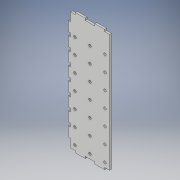
# Autodesk Inventor part: 2 binnen zijplaat
Saved by Autodesk Inventor 2019 (Build 230136000, 136)
## iProperties
Created: 2021-01-09
Part Number: 2 binnen zijplaat
Material: Generic
Document SubType Name: Sheet Metal
Designer: Stefan
Density: 1 g/cm^3
Sheet Metal Rule: Default_mm
Appearance: Default
Author: Stefan
Autodesk Inventor part; units mm, degrees
ref_plane "YZ Plane" through (0, 0, 0) normal (1, 0, 0) x (0, 1, 0)
ref_plane "XZ Plane" through (0, 0, 0) normal (0, 1, 0) x (-1, 0, 0)
ref_plane "XY Plane" through (0, 0, 0) normal (0, 0, 1) x (1, 0, 0)
sketch "Sketch1" plane through (0, 0, 0) normal (0, 0, 1) x (1, 0, 0)
  line L0 (-30, -90.5) -> (30, -90.5)
  line L1 (30, -90.5) -> (30, 90.5)
  line L2 (30, 90.5) -> (-30, 90.5)
  line L3 (-30, 90.5) -> (-30, -90.5)
  line L4 (-30, -90.5) -> (30, 90.5) construction
  line L5 (30, -90.5) -> (-30, 90.5) construction
  circle A0 centre (-23, 60.5) radius 2
  circle A1 centre (-23, 36.5) radius 2
  circle A2 centre (-23, 12.5) radius 2
  circle A3 centre (-23, -11.5) radius 2
  circle A4 centre (-23, -35.5) radius 2
  circle A5 centre (-23, -59.5) radius 2
  circle A6 centre (-23, -83.5) radius 2
  circle A7 centre (0, 60.5) radius 2
  circle A8 centre (0, 36.5) radius 2
  circle A9 centre (0, 12.5) radius 2
  circle A10 centre (0, -11.5) radius 2
  circle A11 centre (0, -35.5) radius 2
  circle A12 centre (0, -59.5) radius 2
  circle A13 centre (0, -83.5) radius 2
  circle A14 centre (23, 60.5) radius 2
  circle A15 centre (23, 36.5) radius 2
  circle A16 centre (23, 12.5) radius 2
  circle A17 centre (23, -11.5) radius 2
  circle A18 centre (23, -35.5) radius 2
  circle A19 centre (23, -59.5) radius 2
  circle A20 centre (23, -83.5) radius 2
  point P0 (0, 0)
  dimension "d0" = 60
  dimension "d1" = 181
  dimension "d2" = 4
  dimension "d3" = 30
  dimension "d6" = 24
  dimension "d9" = 23
  dimension "d12" = 7
  constraints: 21 centre point, 12 end point, 2 horizontal, 2 midpoint, 2 parallel, 1 perpendicular, 1 vertical, 40 other
  measures "d0" distance of L2.end L1.end
  measures "d1" distance of L1.end L0.end
  measures "d2" diameter of A0
  measures "d3" distance from line of A0.centre L2
  measures "d6" distance of A0.centre A1.centre
  measures "d9" distance of A0.centre A7.centre
  measures "d12" distance from line of L3 A0.centre
extrude "Extrusion1" add sketch "Sketch1" along normal blind 3
sketch "Sketch2" plane through (0, 0, 3) normal (0, 0, 1) x (1, 0, 0)
  line L0 (-30, 90.5) -> (-30, -90.5) projected
  line L1 (-30, 77.5) -> (-33, 77.5)
  line L2 (-33, 77.5) -> (-33, 62.5)
  line L3 (-33, 62.5) -> (-30, 62.5)
  line L4 (-30, 62.5) -> (-30, 77.5)
  line L5 (-30, 57.5) -> (-33, 57.5)
  line L6 (-33, 57.5) -> (-33, 42.5)
  line L7 (-33, 42.5) -> (-30, 42.5)
  line L8 (-30, 42.5) -> (-30, 57.5)
  line L9 (-30, 37.5) -> (-33, 37.5)
  line L10 (-33, 37.5) -> (-33, 22.5)
  line L11 (-33, 22.5) -> (-30, 22.5)
  line L12 (-30, 22.5) -> (-30, 37.5)
  line L13 (-30, 17.5) -> (-33, 17.5)
  line L14 (-33, 17.5) -> (-33, 2.5)
  line L15 (-33, 2.5) -> (-30, 2.5)
  line L16 (-30, 2.5) -> (-30, 17.5)
  line L17 (-30, -2.5) -> (-33, -2.5)
  line L18 (-33, -2.5) -> (-33, -17.5)
  line L19 (-33, -17.5) -> (-30, -17.5)
  line L20 (-30, -17.5) -> (-30, -2.5)
  line L21 (-30, -22.5) -> (-33, -22.5)
  line L22 (-33, -22.5) -> (-33, -37.5)
  line L23 (-33, -37.5) -> (-30, -37.5)
  line L24 (-30, -37.5) -> (-30, -22.5)
  line L25 (-30, -42.5) -> (-33, -42.5)
  line L26 (-33, -42.5) -> (-33, -57.5)
  line L27 (-33, -57.5) -> (-30, -57.5)
  line L28 (-30, -57.5) -> (-30, -42.5)
  line L29 (-30, -62.5) -> (-33, -62.5)
  line L30 (-33, -62.5) -> (-33, -77.5)
  line L31 (-33, -77.5) -> (-30, -77.5)
  line L32 (-30, -77.5) -> (-30, -62.5)
  point P0 (0, 0)
  dimension "d15" = 3
  dimension "d16" = 15
  dimension "d17" = 13
  dimension "d20" = 20
  constraints: 64 end point, 2 parallel, 1 horizontal, 1 perpendicular, 1 point on line, 1 vertical, 56 other
  measures "d15" distance of L3.end L2.end
  measures "d16" distance of L2.end L1.end
  measures "d17" distance from line of L0.start L1
  measures "d20" distance of L1.start L5.start
extrude "Extrusion2" add sketch "Sketch2" against normal blind 3
sketch "Sketch3" plane through (0, 0, 3) normal (0, 0, 1) x (1, 0, 0)
  line L0 (30, 90.5) -> (-30, 90.5) projected
  line L1 (-22.5, 90.5) -> (-7.5, 90.5)
  line L2 (-7.5, 90.5) -> (-7.5, 93.5)
  line L3 (-7.5, 93.5) -> (-22.5, 93.5)
  line L4 (-22.5, 93.5) -> (-22.5, 90.5)
  line L5 (-22.5, -93.5) -> (-7.5, -93.5)
  line L6 (-7.5, -93.5) -> (-7.5, -90.5)
  line L7 (-7.5, -90.5) -> (-22.5, -90.5)
  line L8 (-22.5, -90.5) -> (-22.5, -93.5)
  line L9 (7.5, 90.5) -> (22.5, 90.5)
  line L10 (22.5, 90.5) -> (22.5, 93.5)
  line L11 (22.5, 93.5) -> (7.5, 93.5)
  line L12 (7.5, 93.5) -> (7.5, 90.5)
  line L13 (7.5, -93.5) -> (22.5, -93.5)
  line L14 (22.5, -93.5) -> (22.5, -90.5)
  line L15 (22.5, -90.5) -> (7.5, -90.5)
  line L16 (7.5, -90.5) -> (7.5, -93.5)
  line L17 (-30, 90.5) -> (-30, 77.5) projected
  point P0 (0, 0)
  dimension "d27" = 15
  dimension "d28" = 3
  dimension "d31" = 184
  dimension "d34" = 30
  dimension "d37" = 7.5
  constraints: 32 end point, 2 collinear, 2 horizontal, 2 parallel, 1 perpendicular, 1 point on line, 1 vertical, 22 other
  measures "d27" distance of L3.end L2.end
  measures "d28" distance of L2.end L1.end
  measures "d31" distance of L1.start L5.start
  measures "d34" distance of L1.start L9.start
  measures "d37" distance between parallel lines of L17 L4
extrude "Extrusion3" add sketch "Sketch3" against normal blind 3
equation "\"BendRadius\" = Thickness"
equation "\"BendReliefWidth\" = Thickness"
equation "\"BendReliefDepth\" = 0.5 * Thickness"
equation "\"CornerReliefSize\" = 4 * Thickness"
equation "\"MinimumRemnant\" = 2 * Thickness"
equation "\"TransitionRadius\" = BendRadius"
equation "\"JacobiRadiusSize\" = BendRadius"
equation "\"GapSize\" = Thickness"
equation "\"Thickness\" = 0.5"
body "Solid1"
